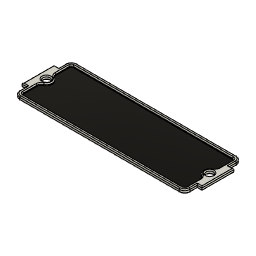
gridfinity_label_parametric v11 (Autodesk Fusion 360 design; units mm, degrees)
Autodesk Fusion 360 part; units mm, degrees
note: some values were not read from the file. Set by a fixed rule: which sketch regions a step uses.
sketch "Sketch1" plane through (0, 0, 35.65) normal (0, 0, 1) x (-1, 0, 0)
  line L0 (-2.15, 2.65) -> (-18.9, 2.65)
  line L1 (-0.25, -3.35) -> (-0.25, -0.5)
  line L2 (-1.25, -0.5) -> (-1.25, 1.5)
  arc A0 (-1.25, 1.5) -> (-2.15, 2.4) centre (-2.15, 1.5) ccw
  line L3 (-2.15, 2.4) -> (-18.9, 2.4)
  line L4 (-1.25, -0.5) -> (-0.25, -0.5)
  line L5 (0, -3.35) -> (0, 0)
  line L6 (0, 0) -> (-1, 0)
  line L7 (-1, 0) -> (-1, 1.5)
  arc A1 (-1, 1.5) -> (-2.15, 2.65) centre (-2.15, 1.5) ccw
  line L8 (-18.9, -3.35) -> (-18.9, 2.65)
  line L9 (0, -3.35) -> (-18.9, -3.35)
  line L10 (0, 0) -> (-24, 0) construction
  line L11 (0, -3.35) -> (0, -6.7)
  line L12 (-1, -6.7) -> (-1, -8.2)
  line L13 (0, -3.35) -> (-18.9, -3.35)
  line L14 (-1.25, -6.2) -> (-0.25, -6.2)
  arc A2 (-2.15, -9.35) -> (-1, -8.2) centre (-2.15, -8.2) ccw
  line L15 (-2.15, -9.35) -> (-18.9, -9.35)
  line L16 (-1.25, -6.2) -> (-1.25, -8.2)
  line L17 (0, -6.7) -> (-1, -6.7)
  arc A3 (-2.15, -9.1) -> (-1.25, -8.2) centre (-2.15, -8.2) ccw
  line L18 (-0.25, -3.35) -> (-0.25, -6.2)
  line L19 (-2.15, -9.1) -> (-18.9, -9.1)
  line L20 (-18.9, -3.35) -> (-18.9, -9.35)
  line L21 (-36.55, -6.2) -> (-37.55, -6.2)
  line L22 (-37.8, -6.7) -> (-36.8, -6.7)
  line L23 (-35.65, -9.35) -> (-18.9, -9.35)
  line L24 (-37.8, -3.35) -> (-18.9, -3.35)
  line L25 (-36.8, 0) -> (-36.8, 1.5)
  line L26 (-35.65, 2.4) -> (-18.9, 2.4)
  line L27 (-36.55, -0.5) -> (-37.55, -0.5)
  line L28 (-35.65, 2.65) -> (-18.9, 2.65)
  arc A4 (-35.65, 2.4) -> (-36.55, 1.5) centre (-35.65, 1.5) ccw
  line L29 (-37.55, -3.35) -> (-37.55, -6.2)
  line L30 (-37.55, -3.35) -> (-37.55, -0.5)
  line L31 (-37.8, -3.35) -> (-18.9, -3.35)
  line L32 (-36.55, -6.2) -> (-36.55, -8.2)
  arc A5 (-36.55, -8.2) -> (-35.65, -9.1) centre (-35.65, -8.2) ccw
  line L33 (-37.8, -3.35) -> (-37.8, 0)
  line L34 (-18.9, -3.35) -> (-18.9, 2.65)
  line L35 (-37.8, 0) -> (-36.8, 0)
  arc A6 (-35.65, 2.65) -> (-36.8, 1.5) centre (-35.65, 1.5) ccw
  arc A7 (-36.8, -8.2) -> (-35.65, -9.35) centre (-35.65, -8.2) ccw
  line L36 (-36.55, -0.5) -> (-36.55, 1.5)
  line L37 (-35.65, -9.1) -> (-18.9, -9.1)
  line L38 (-36.8, -6.7) -> (-36.8, -8.2)
  line L39 (-18.9, -3.35) -> (-18.9, -9.35)
  line L40 (-37.8, -3.35) -> (-37.8, -6.7)
  point P0 (0, -6.7)
  point P1 (0, -6.7)
  point P2 (-37.8, -6.7)
  point P3 (-37.8, -6.7)
  point P4 (-37.8, 0)
  point P5 (-37.8, 0)
  dimension "d562" = 0.25
  dimension "d566" = 0.5
  dimension "d4" = 18.9
  dimension "d5" = 3.35
  dimension "d6" = 1
  dimension "d7" = 1
  dimension "d8" = 1.15
  dimension "d9" = 0.9
  dimension "d10" = 2
  dimension "d11" = 1.5
  dimension "d12" = 0.9
  dimension "d13" = 1.15
  constraint coincident L1 L4.end
  constraint perpendicular L1 L4
  constraint tangent L2 A0
  constraint tangent A0 L3
  constraint coincident A0.centre A1.centre
  constraint coincident L5.end L6.start
  constraint coincident L8 L3.end
  constraint coincident L9 L1.start
  constraint parallel L0 L3
  constraint perpendicular L6 L7
  constraint perpendicular L5 L9
  constraint parallel L9 L10
  constraint symmetric L5.end L9 P1
  constraint symmetric L0.start L9 A2.start
  constraint symmetric L2.end L9 L16.end
  constraint symmetric A0.end L9 A3.start
  constraint symmetric A0 L9 A3
  constraint symmetric L2.start L9 L14.start
  constraint symmetric L1.end L9 L14.end
  constraint symmetric L6.end L9 L12.start
  constraint symmetric L7.end L9 L12.end
  constraint symmetric A1 L9 A2
  constraint symmetric L5.start L9 L11.start
  constraint symmetric L8.start L9 L13.end
  constraint symmetric L0.end L9 L15.end
  constraint symmetric L3.end L9 L19.end
  constraint symmetric L9 L1.start L18.start
  constraint symmetric L9 L5.end P1
  constraint symmetric L5.end L20 P5
  constraint symmetric L0.start L20 L28.start
  constraint symmetric L2.end L20 A4.end
  constraint symmetric A0.end L20 L26.start
  constraint symmetric A0 L20 A4
  constraint symmetric L2.start L20 L27.start
  constraint symmetric L1.end L20 L27.end
  constraint symmetric L6.end L20 L25.start
  constraint symmetric L7.end L20 L25.end
  constraint symmetric A1 L20 A6
  constraint symmetric L5.start L20 L24.start
  constraint symmetric L8.start L20 L9.end
  constraint symmetric L0.end L20 L8.end
  constraint symmetric L3.end L20 L26.end
  constraint symmetric L1.start L20 L29.start
  constraint symmetric L15.end L20 L23.end
  constraint symmetric A3.start L20 A5.end
  constraint symmetric L12.end L20 A7.start
  constraint symmetric P1 L20 P3
  constraint symmetric L12.start L20 L22.end
  constraint symmetric L19.end L20 L37.end
  constraint symmetric L16.end L20 L32.end
  constraint symmetric L14.end L20 L21.end
  constraint symmetric A2.start L20 L23.start
  constraint symmetric L14.start L20 L21.start
  constraint symmetric A2 L20 A7
  constraint symmetric A3 L20 A5
  constraint perpendicular L3 L34
  measures "d562" distance of L1 L5
  measures "d566" distance of L4 L6
  measures "d4" distance of L5.start L8.start
  measures "d5" distance of L5.end L5.start
  measures "d6" distance of L5.end L6.end
  measures "d7" distance of L2.start L1.end
  measures "d8" radius of A1
  measures "d9" radius of A0
  measures "d10" distance of L2.end L2.start
  measures "d11" distance of L6.end L7.end
  measures "d12" distance of L2 A0.end
  measures "d13" horizontal distance of L0.start L7.end
extrude "Extrude1" add sketch "Sketch1" along normal blind 0.4
sketch "Sketch2" plane through (0, 0, 36.05) normal (0, 0, 1) x (-1, 0, 0)
  line L0 (-2.15, -8.6) -> (-35.65, -8.6)
  line L1 (-36.05, -8.2) -> (-36.05, 1.5)
  line L2 (-35.65, 1.9) -> (-2.15, 1.9)
  line L3 (-1.75, 1.5) -> (-1.75, -8.2)
  arc A0 (-2.15, -8.6) -> (-1.75, -8.2) centre (-2.15, -8.2) ccw
  arc A1 (-1.75, 1.5) -> (-2.15, 1.9) centre (-2.15, 1.5) ccw
  arc A2 (-35.65, 1.9) -> (-36.05, 1.5) centre (-35.65, 1.5) ccw
  arc A3 (-36.05, -8.2) -> (-35.65, -8.6) centre (-35.65, -8.2) ccw
  circle A4 centre (-1.75, -3.35) radius 0.75
  circle A5 centre (-36.05, -3.35) radius 0.75
  circle A6 centre (-1.75, -3.35) radius 1.25
  circle A7 centre (-36.05, -3.35) radius 1.25
  arc A8 (-2.15, -9.35) -> (-1, -8.2) centre (-2.15, -8.2) ccw
  line L4 (-1, -8.2) -> (-1, -6.7)
  line L5 (-1, -6.7) -> (0, -6.7)
  line L6 (0, -6.7) -> (0, 0)
  line L7 (0, 0) -> (-1, 0)
  line L8 (-1, 0) -> (-1, 1.5)
  arc A9 (-1, 1.5) -> (-2.15, 2.65) centre (-2.15, 1.5) ccw
  arc A10 (-35.65, 2.65) -> (-36.8, 1.5) centre (-35.65, 1.5) ccw
  line L9 (-2.15, 2.65) -> (-35.65, 2.65)
  arc A11 (-35.65, 2.65) -> (-36.8, 1.5) centre (-35.65, 1.5) ccw
  line L10 (-36.8, 1.5) -> (-36.8, 0)
  line L11 (-36.8, 0) -> (-37.8, 0)
  line L12 (-37.8, 0) -> (-37.8, -6.7)
  line L13 (-37.8, -6.7) -> (-36.8, -6.7)
  line L14 (-36.8, -6.7) -> (-36.8, -8.2)
  arc A12 (-36.8, -8.2) -> (-35.65, -9.35) centre (-35.65, -8.2) ccw
  line L15 (-35.65, -9.35) -> (-2.15, -9.35)
  point P0 (-2.15, -8.2)
  dimension "d517" = 1.5
  dimension "d518" = 2.5
  constraint horizontal L0
  constraint vertical L1
  constraint horizontal L2
  constraint vertical L3
  constraint tangent L0 A0
  constraint tangent L3 A0
  constraint tangent L3 A1
  constraint tangent L2 A1
  constraint equal A0 A1
  constraint tangent L2 A2
  constraint tangent L1 A2
  constraint equal A0 A2
  constraint tangent L1 A3
  constraint tangent L0 A3
  constraint equal A0 A3
  constraint midpoint L3 A4.centre
  constraint midpoint L1 A5.centre
  constraint concentric A4 A6
  constraint concentric A5 A7
  constraint equal A4 A5
  constraint equal A6 A7
  constraint coincident P0 A0.centre
  constraint concentric A2 A10
  measures "d517" diameter of A4
  measures "d518" diameter of A6
extrude "Extrude2" add sketch "Sketch2" along normal blind 0.4 contours L3 A4 A6 | L3 A4 A6 | L1 A5 A7 | L1 A5 A7 | L3 A4 | L3 A4 | L1 A5 | L1 A5 | A8 L4 L5 L6 L7 L8 A9 A10 L9 A11 L10 L11 L12 L13 L14 A12 L15
fillet "Fillet2" radius 1 4 edges at (1.75, 2.1, 36.25) (1.75, 4.6, 36.25) (36.05, 2.1, 36.25) (36.05, 4.6, 36.25)
extrude "Extrude4" cut sketch "Sketch2" along normal through all and the other way through all contours L3 A4 | L3 A4 | L1 A5 | L1 A5
fillet "Fillet1" radius 0.2 2 faces at (37.4667, 3.35, 36.45) (18.9, 1.35, 35.65)
equation "d525 = 0.0 °"
equation "d4 = ( 37.8 / 2 ) * 1 mm + ( ( bin_span - 1 ) * 42 / 2 ) * 1 mm"
equation "bin_span = 1" comment "How many Gridfinity grid swaures does the label span."
equation "picto_inner_diameter = 1 mm"
equation "picto_outer_diameter = 1 mm"
equation "picto_inner_length = 1 mm"
equation "picto_outer_length = 1 mm"
equation "label_text = 0" comment "[label_text]"
equation "gla_id = 0" comment "gridfinity-label-autogen-label"
